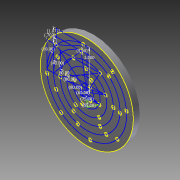
# Autodesk Inventor part: dishConfig
Saved by Autodesk Inventor 2012 (Build 160160000, 160)
## iProperties
Created: 2012-07-31
Part Number: dishConfig
Material: Default
Document SubType Name: Modeling
Designer: Administrator
Density: 1 g/cm^3
Author: Administrator
Autodesk Inventor part; units mm, degrees
ref_plane "YZ Plane" through (0, 0, 0) normal (1, 0, 0) x (0, 1, 0)
ref_plane "XZ Plane" through (0, 0, 0) normal (0, 1, 0) x (-1, 0, 0)
ref_plane "XY Plane" through (0, 0, 0) normal (0, 0, 1) x (1, 0, 0)
sketch "Sketch3" plane through (0, 0, 0) normal (0, 0, 1) x (1, 0, 0)
  circle A0 centre (0, 0) radius 12.7
  circle A1 centre (0, 0) radius 25.4
  circle A2 centre (0, 0) radius 38.1
  circle A3 centre (0, 0) radius 50.8
  circle A4 centre (0, 0) radius 63.5
  circle A5 centre (0, 0) radius 76.2
  line L0 (0, 0) -> (-12.7, 0)
  line L1 (0, 0) -> (-58.3726, 48.9804)
  line L2 (0, 0) -> (-11.0267, 62.5353)
  line L3 (0, 0) -> (25.4, 43.9941)
  line L4 (0, 0) -> (35.8023, 13.031)
  line L5 (0, 0) -> (23.8682, -8.6873)
  line L6 (23.8682, -8.6873) -> (0, 0)
  line L7 (0, 0) -> (-75.91, -6.6413)
  line L8 (0, 0) -> (-48.9804, -58.3726)
  line L9 (0, 0) -> (6.6413, -75.91)
  line L10 (0, 0) -> (58.3726, -48.9804)
  line L11 (0, 0) -> (75.91, 6.6413)
  line L12 (0, 0) -> (48.9804, 58.3726)
  line L13 (0, 0) -> (-6.6413, 75.91)
  line L14 (0, 0) -> (-55.7671, 30.3691)
  line L15 (0, 0) -> (-58.5137, -24.6656)
  line L16 (0, 0) -> (-17.1984, -61.1266)
  line L17 (0, 0) -> (37.0677, -51.5581)
  line L18 (0, 0) -> (63.4211, -3.1652)
  line L19 (0, 0) -> (42.0171, 47.6111)
  line L20 (0, 0) -> (-25.4, 43.9941)
  line L21 (0, 0) -> (-50.8, 0)
  line L22 (0, 0) -> (-25.4, -43.9941)
  line L23 (0, 0) -> (25.4, -43.9941)
  line L24 (0, 0) -> (50.8, 0)
  line L25 (0, 0) -> (-1.3297, 38.0768)
  line L26 (0, 0) -> (-36.6241, 10.5018)
  line L27 (0, 0) -> (-21.3052, -31.5863)
  line L28 (0, 0) -> (23.4567, -30.0232)
  line L29 (0, 0) -> (8.6873, 23.8682)
  line L30 (0, 0) -> (-23.8682, 8.6873)
  line L31 (0, 0) -> (-8.6873, -23.8682)
  line L32 (0, 0) -> (6.35, -10.9985)
  line L33 (0, 0) -> (6.35, 10.9985)
  circle A6 centre (0, 0) radius 88.9
  dimension "d104" = 12.7
  dimension "d105" = 12.7
  dimension "d106" = 12.7
  dimension "d107" = 12.7
  dimension "d108" = 12.7
  dimension "d110" = 25.4
  dimension "d111" = 40
  dimension "d112" = 40
  dimension "d113" = 40
  dimension "d114" = 40
  dimension "d115" = 40
  dimension "d118" = 360
  dimension "d122" = 360
  dimension "d126" = 360
  dimension "d130" = 360
  dimension "d134" = 360
  dimension "d138" = 360
  dimension "d140" = 12.7
  constraints: 68 end point, 42 coincident, 1 centre point, 1 collinear, 1 horizontal, 1 horizontal alignment, 153 other
  measures "d111" angle of L0 L1
  measures "d112" angle of L2 L1
  measures "d113" angle of L2 L3
  measures "d114" angle of L3 L4
  measures "d115" angle of L4 L5
extrude "Extrusion3" add sketch "Sketch3" along normal blind 12.7 contours L24 L11 A0 | L24 A1 L18 A0 | A0 L18 L24 | A0 L11 A1 L24 | L11 L4 A0 | A0 L4 A1 L11 | L18 A1 L5 A0 | A0 L5 L18 | L7 A0 L0 | L14 A0 L1 | L20 A0 L2 | L29 A0 L3 | L19 A0 L4 | L15 A0 L7 | L27 A0 L8 | L23 A0 L9 | L5 A0 L10 | L3 A0 L12 | L2 A0 L13 | L30 A0 L14 | L8 A0 L15 | L9 A0 L16 | L28 A0 L17 | L12 A0 L19 | L1 A0 L20 | L31 A0 L22 | L17 A0 L23 | L13 A0 L25 | L0 A0 L26 | L22 A0 L27 | L10 A0 L28 | L25 A0 L29 | L26 A0 L30 | L16 A0 L31 | L24 A2 L18 A1 | A1 L11 A2 L24 | A0 L19 A1 L4 | A1 L4 A2 L11 | L5 A1 L10 A0 | L18 A2 L10 A1 | L21 A1 L26 A0 | A0 L7 A1 L21 | L1 A1 L20 A0 | A0 L14 A1 L1 | L2 A1 L13 A0 | A0 L20 A1 L2 | L3 A1 L12 A0 | A0 L29 A1 L3 | A0 L15 A1 L7 | L8 A1 L15 A0 | A0 L27 A1 L8 | L9 A1 L16 A0 | A0 L23 A1 L9 | L10 A1 L28 A0 | L12 A1 L19 A0 | L13 A1 L25 A0 | A0 L30 A1 L14 | L16 A1 L31 A0 | L17 A1 L23 A0 | A0 L28 A1 L17 | L22 A1 L27 A0 | A0 L31 A1 L22 | L25 A1 L29 A0 | L26 A1 L30 A0 | L24 A3 L18 A2 | A2 L11 A3 L24 | A1 L19 A2 L4 | A2 L19 A3 L11 | L18 A3 L10 A2 | L21 A2 L26 A1 | A1 L7 A2 L21 | L1 A2 L20 A1 | A1 L14 A2 L1 | L2 A2 L13 A1 | A1 L20 A2 L2 | L3 A2 L12 A1 | A1 L25 A2 L3 | A1 L15 A2 L7 | L8 A2 L15 A1 | A1 L27 A2 L8 | L9 A2 L16 A1 | A1 L23 A2 L9 | L10 A2 L28 A1 | L12 A2 L19 A1 | L13 A2 L25 A1 | A1 L26 A2 L14 | L16 A2 L22 A1 | L17 A2 L23 A1 | A1 L28 A2 L17 | L22 A2 L27 A1 | A3 L11 A4 L18 | A3 L19 A4 L11 | L10 A3 L17 A2 | L18 A4 L10 A3 | L21 A3 L14 A2 | A2 L7 A3 L21 | L1 A3 L20 A2 | A2 L14 A3 L1 | L2 A3 L13 A2 | A2 L20 A3 L2 | L3 A3 L12 A2 | A2 L13 A3 L3 | A2 L15 A3 L7 | L8 A3 L15 A2 | A2 L22 A3 L8 | L9 A3 L16 A2 | A2 L23 A3 L9 | L12 A3 L19 A2 | L16 A3 L22 A2 | L17 A3 L23 A2 | A3 L12 A4 L19 | L11 A5 L10 A4 | A4 L12 A5 L11 | L10 A4 L17 A3 | A3 L7 A4 L14 | L1 A4 L2 A3 | A3 L14 A4 L1 | L2 A4 L13 A3 | A3 L13 A4 L12 | A3 L15 A4 L7 | L8 A4 L15 A3 | A3 L16 A4 L8 | L9 A4 L16 A3 | A3 L17 A4 L9 | L10 A5 L9 A4 | L1 A5 L13 A4 | A4 L7 A5 L1 | A4 L8 A5 L7 | A4 L9 A5 L8 | A4 L13 A5 L12 | A6
hole "Hole2" at (-58.3726, 48.9804, 0) at (-11.0267, 62.5353, 0) at (25.4, 43.9941, 0) at (35.8023, 13.031, 0) at (23.8682, -8.6873, 0) at (-12.7, 0, 0) at (-75.91, -6.6413, 0) at (-48.9804, -58.3726, 0) at (6.6413, -75.91, 0) at (58.3726, -48.9804, 0) at (75.91, 6.6413, 0) at (48.9804, 58.3726, 0) at (-6.6413, 75.91, 0) at (-55.7671, 30.3691, 0) at (-58.5137, -24.6656, 0) at (-17.1984, -61.1266, 0) at (37.0677, -51.5581, 0) at (63.4211, -3.1652, 0) at (42.0171, 47.6111, 0) at (-25.4, 43.9941, 0) at (-50.8, 0, 0) at (-25.4, -43.9941, 0) at (25.4, -43.9941, 0) at (50.8, 0, 0) at (-1.3297, 38.0768, 0) at (-36.6241, 10.5018, 0) at (-21.3052, -31.5863, 0) at (23.4567, -30.0232, 0) at (8.6873, 23.8682, 0) at (-23.8682, 8.6873, 0) at (-8.6873, -23.8682, 0) at (6.35, -10.9985, 0) at (6.35, 10.9985, 0) direction (0, 0, 1) diameter 6.35 end through all
sketch "Sketch5" plane through (0, 0, 12.7) normal (0, 0, 1) x (1, 0, 0)
  circle A0 centre (6.35, 10.9985) radius 3.175 projected
  circle A1 centre (6.35, -10.9985) radius 3.175 projected
  circle A2 centre (-8.6873, -23.8682) radius 3.175 projected
  circle A3 centre (-23.8682, 8.6873) radius 3.175 projected
  circle A4 centre (8.6873, 23.8682) radius 3.175 projected
  circle A5 centre (23.4567, -30.0232) radius 3.175 projected
  circle A6 centre (-21.3052, -31.5863) radius 3.175 projected
  circle A7 centre (-36.6241, 10.5018) radius 3.175 projected
  circle A8 centre (-1.3297, 38.0768) radius 3.175 projected
  circle A9 centre (50.8, 0) radius 3.175 projected
  circle A10 centre (25.4, -43.9941) radius 3.175 projected
  circle A11 centre (-25.4, -43.9941) radius 3.175 projected
  circle A12 centre (-50.8, 0) radius 3.175 projected
  circle A13 centre (-25.4, 43.9941) radius 3.175 projected
  circle A14 centre (42.0171, 47.6111) radius 3.175 projected
  circle A15 centre (63.4211, -3.1652) radius 3.175 projected
  circle A16 centre (37.0677, -51.5581) radius 3.175 projected
  circle A17 centre (-17.1984, -61.1266) radius 3.175 projected
  circle A18 centre (-58.5137, -24.6656) radius 3.175 projected
  circle A19 centre (-55.7671, 30.3691) radius 3.175 projected
  circle A20 centre (-6.6413, 75.91) radius 3.175 projected
  circle A21 centre (48.9804, 58.3726) radius 3.175 projected
  circle A22 centre (75.91, 6.6413) radius 3.175 projected
  circle A23 centre (58.3726, -48.9804) radius 3.175 projected
  circle A24 centre (6.6413, -75.91) radius 3.175 projected
  circle A25 centre (-48.9804, -58.3726) radius 3.175 projected
  circle A26 centre (-75.91, -6.6413) radius 3.175 projected
  circle A27 centre (-12.7, 0) radius 3.175 projected
  circle A28 centre (23.8682, -8.6873) radius 3.175 projected
  circle A29 centre (35.8023, 13.031) radius 3.175 projected
  circle A30 centre (25.4, 43.9941) radius 3.175 projected
  circle A31 centre (-11.0267, 62.5353) radius 3.175 projected
  circle A32 centre (-58.3726, 48.9804) radius 3.175 projected
  circle A33 centre (0, 0) radius 88.9 projected
  line L0 (0, 0) -> (-58.3726, 48.9804)
  line L1 (0, 0) -> (-11.0267, 62.5353)
  line L2 (0, 0) -> (25.4, 43.9941)
  line L3 (0, 0) -> (35.8023, 13.031)
  line L4 (0, 0) -> (23.8682, -8.6873)
  line L5 (0, 0) -> (6.35, -10.9985)
  line L6 (0, 0) -> (-76.2, 0)
  circle A34 centre (0, 0) radius 12.7
  circle A35 centre (0, 0) radius 25.4
  circle A36 centre (0, 0) radius 38.1
  circle A37 centre (0, 0) radius 50.8
  circle A38 centre (0, 0) radius 63.5
  circle A39 centre (0, 0) radius 76.2
  line L7 (-76.2, 0) -> (-76.2, 48.9804)
  line L8 (-76.2, 48.9804) -> (-58.3726, 48.9804)
  line L9 (-76.2, 0) -> (-58.3726, 48.9804)
  line L10 (-63.5, 0) -> (-63.5, 62.5353)
  line L11 (-63.5, 62.5353) -> (-11.0267, 62.5353)
  line L12 (-63.5, 0) -> (-11.0267, 62.5353)
  line L13 (25.4, 43.9941) -> (-50.8, 43.9941)
  line L14 (-50.8, 43.9941) -> (-50.8, 0)
  line L15 (-50.8, 0) -> (25.4, 43.9941)
  line L16 (35.8023, 13.031) -> (-38.1, 13.031)
  line L17 (-38.1, 13.031) -> (-38.1, 0)
  line L18 (35.8023, 13.031) -> (-38.1, 0)
  line L19 (-25.4, 0) -> (-25.4, -8.6873)
  line L20 (-25.4, -8.6873) -> (23.8682, -8.6873)
  line L21 (-25.4, 0) -> (23.8682, -8.6873)
  line L22 (-12.7, 0) -> (-12.7, -10.9985)
  line L23 (-12.7, -10.9985) -> (6.35, -10.9985)
  line L24 (-12.7, 0) -> (6.35, -10.9985)
  line L25 (-58.3726, 48.9804) -> (0, 76.2)
  line L26 (0, -25.4) -> (0, -8.6873)
  line L27 (23.8682, -8.6873) -> (0, -25.4)
  line L28 (0, -12.7) -> (0, -10.9985)
  line L29 (0, -12.7) -> (6.35, -10.9985)
  line L30 (0, 76.2) -> (-58.3726, 76.2)
  line L31 (-58.3726, 76.2) -> (-58.3726, 48.9804)
  line L32 (0, 63.5) -> (-11.0267, 63.5)
  line L33 (-11.0267, 63.5) -> (-11.0267, 62.5353)
  line L34 (-11.0267, 62.5353) -> (0, 63.5)
  line L35 (0, 76.2) -> (0, 0)
  dimension "d155" = 20
  dimension "d156" = 40
  dimension "d157" = 60
  dimension "d158" = 80
  dimension "d159" = 80
  dimension "d160" = 60
  dimension "d161" = 76.2
  dimension "d172" = 55
  dimension "d173" = 75
  dimension "d174" = 5
  dimension "d175" = 27.2196
  dimension "d176" = 17.8274
  constraints: 72 end point, 14 point on circle, 11 perpendicular, 8 point on line, 6 coincident, 6 tangent, 5 centre point, 3 horizontal, 3 parallel, 2 vertical, 1 midpoint, 3 other
  measures "d155" angle of L9 L7
  measures "d156" angle of L10 L12
  measures "d157" angle of L15 L14
  measures "d158" angle of L18 L17
  measures "d159" angle of L21 L19
  measures "d160" angle of L24 L22
  measures "d161" distance of L0.start L25.end
  measures "d172" angle of L27 L26
  measures "d173" angle of L28 L29
  measures "d174" angle of L34 L32
  measures "d175" distance of L30.end L0.end
  measures "d176" distance of L7.end L0.end
equation "\"d112\" = d111"
equation "\"d113\" = d111"
equation "\"d114\" = d111"
equation "\"d115\" = d111"
body "Solid3"
